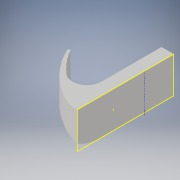
# Autodesk Inventor part: main_front
Saved by Autodesk Inventor 2019 (Build 230136000, 136)
## iProperties
Created: 2019-02-22
Part Number: main_front
Material: Generic
Document SubType Name: Modeling
Designer: gaincarlo
Density: 1 g/cm^3
Appearance: Default
Author: gaincarlo
Autodesk Inventor part; units mm, degrees
ref_plane "YZ Plane" through (0, 0, 0) normal (1, 0, 0) x (0, 1, 0)
sketch "Sketch1" plane through (0, 0, 0) normal (0, 1, 0) x (-1, 0, 0)
  arc A0 (1485.6726, 459.6267) -> (500, 0) centre (1100, 0) ccw
  arc A1 (750, 1299.0381) -> (0, 1500) centre (0, 0) ccw
  line L0 (0, 1500) -> (0, -2500)
  line L1 (0, 0) -> (500, 0) construction
  line L2 (0, 0) -> (4307.852, 0) construction
  arc A2 (2375.2311, -474.5905) -> (750, 1299.0381) centre (-1250, -2165.0635) ccw
  line L3 (0, 0) -> (750, 1299.0381) construction
  line L4 (2533.8122, -814.6686) -> (2153.926, 0) construction
  line L5 (500, 0) -> (500, -2500)
  line L6 (1100, 0) -> (1485.6726, 459.6267) construction
  arc A3 (2286.5935, -515.9229) -> (1485.6726, 459.6267) centre (-716.704, -2165.0635) ccw
  line L7 (2375.2311, -474.5905) -> (2286.5935, -515.9229)
  line L8 (-1250, -2165.0635) -> (1570, -2165.0635) construction
  line L9 (500, -2500) -> (0, -2500)
  dimension "d0" = 1200
  dimension "d1" = 3000
  dimension "d3" = 500
  dimension "d4" = 4000
  dimension "d5" = 30
  dimension "d6" = 25
  dimension "d7" = 40
  dimension "d9" = 3426.2897
  dimension "d10" = 2500
  constraints: 20 end point, 9 point on circle, 4 centre point, 4 point on line, 3 horizontal, 3 tangent, 2 coincident, 2 perpendicular, 2 vertical, 1 midpoint
  measures "d0" diameter of A0
  measures "d1" diameter of A1
  measures "d3" distance from line of L1.end L0
  measures "d4" radius of A2
  measures "d5" angle of L0 L3
  measures "d6" angle of L4 L0
  measures "d7" angle of L5 L6
  measures "d9" radius of A3
  measures "d10" distance of L1.end L5.end
extrude "Extrusion1" add sketch "Sketch1" along normal mid plane 1500
sketch "Sketch3" plane through (0, -750, 0) normal (0, -1, 0) x (1, 0, 0)
  line L0 (0, -1289.8041) -> (-2443.3584, 421.0539) construction
  arc A0 (-750, 1299.0381) -> (-2375.2311, -474.5905) centre (1250, -2165.0635) ccw construction
  line L1 (0, -2500) -> (0, 1500) projected
  point P0 (0, 0)
  dimension "d15" = 55
  constraints: 2 end point, 1 line through centre, 1 point on line
  measures "d15" angle of L1 L0
sketch "Sketch2" plane through (0, -750, -2500) normal (1, 0, 0) x (0, 0, -1)
  line L0 (0, 0) -> (0, 1500) construction
  line L1 (-4000, 1500) -> (0, 1500) construction
  line L2 (-4000, 1500) -> (-4000, 0) construction
  line L3 (0, 0) -> (-4000, 0) construction
  line L4 (-3000, 0) -> (-3000, 1500) construction
  line L5 (0, 0) -> (-4000, 0) projected
  arc A0 (-4566.8639, 757.0449) -> (-3000, 0) centre (-3000, 2000) ccw
  line L6 (-3000, 0) -> (-3000, -688)
  line L7 (-3000, -688) -> (-5471, 267.9492)
  line L8 (-5471, 267.9492) -> (-4566.8639, 757.0449)
  point P0 (-2500, 750)
  dimension "d13" = 1000
  dimension "d14" = 4000
  constraints: 8 end point, 3 point on line, 2 point on circle, 1 centre point, 1 perpendicular, 1 tangent, 1 vertical
  measures "d13" distance between parallel lines of L2 L4
  measures "d14" diameter of A0
ref_plane "Work Plane2" through (0, 750, -915) normal (-0.7071, 0, -0.7071) x (0, -1, 0)
sketch "Sketch4" plane through (0, -750, -2500) normal (1, 0, 0) x (0, 0, -1)
  line L0 (0, 0) -> (-4000, 0) projected
  line L1 (-4000, 0) -> (-4000, 1500) projected
  line L2 (-4000, 1500) -> (0, 1500) projected
  line L3 (0, 1500) -> (0, 0) projected
  line L4 (0, 0) -> (-4000, 0) projected
  line L5 (-4000, 0) -> (-4000, 1500) projected
  line L6 (-4000, 1500) -> (0, 1500) projected
  line L7 (0, 1500) -> (0, 0) projected
  line L8 (-1210.1959, 0) -> (-2921.0539, 0) construction
  line L9 (0, 0) -> (-4000, 0) projected
  line L10 (-1210.1959, 0) -> (-1210.1959, 1500) construction
  point P0 (-2500, 750)
  constraints: 2 end point, 1 coincident, 1 perpendicular, 1 point on line
ref_plane "Work Plane3" through (0, 750, -1289.8041) normal (-0.5736, 0, -0.8192) x (0, -1, 0)
sketch "Sketch7" plane through (0, 750, -1289.8041) normal (-0.5736, 0, -0.8192) x (0, -1, 0)
  arc A0 (1500, 2323.4905) -> (1202.693, 2568.9738) centre (1250, 2323.4905) ccw
  line L0 (1500, 0) -> (1500, 2982.7898) construction
  line L1 (1500, 2474.0318) -> (1500, 2323.4905) construction
  line L2 (1500, 2323.4905) -> (0, 2323.4905) construction
  line L3 (0, 2323.4905) -> (0, 2474.0318) construction
  line L4 (0, 2474.0318) -> (1500, 2474.0318) construction
  line L5 (1500, 610.3873) -> (1500, 0) construction
  line L6 (1500, 0) -> (0, 0) construction
  line L7 (0, 0) -> (0, 610.3873) construction
  line L8 (0, 610.3873) -> (1500, 610.3873) construction
  line L9 (1202.693, 2568.9738) -> (1046, 3413)
  line L10 (1046, 3413) -> (2457, 2027)
  line L11 (2457, 2027) -> (1500, 2323.4905)
  point P0 (750, 739.8012)
  dimension "d34" = 500
  constraints: 6 end point, 3 point on circle, 1 centre point, 1 point on line, 1 tangent
  measures "d34" diameter of A0
loft "Loft5" cut profiles "Sketch2", "Sketch7"
body "Solid1"
